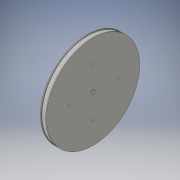
# Autodesk Inventor part: Wheel
Saved by Autodesk Inventor 2016 (Build 200138000, 138)
## iProperties
Created: 2016-10-07
Part Number: Wheel
Material: Generic
Document SubType Name: Modeling
Designer: sheehm
Density: 1 g/cm^3
Appearance: Default
Author: sheehm
Autodesk Inventor part; units mm, degrees
ref_plane "YZ Plane" through (0, 0, 0) normal (1, 0, 0) x (0, 1, 0)
ref_plane "XZ Plane" through (0, 0, 0) normal (0, 1, 0) x (-1, 0, 0)
ref_plane "XY Plane" through (0, 0, 0) normal (0, 0, 1) x (1, 0, 0)
sketch "Sketch1" plane through (0, 0, 0) normal (1, 0, 0) x (0, 1, 0)
  circle A0 centre (0, 0) radius 30.48
  dimension "d0" = 60.96
  constraints: 1 centre point, 1 coincident
  measures "d0" diameter of A0
extrude "Extrusion1" add sketch "Sketch1" along normal blind 3.048
sketch "Sketch2" plane through (3.048, 0, 0) normal (1, 0, 0) x (0, 0, -1)
  circle A0 centre (0, 0) radius 30.9541
  constraints: 1 centre point, 1 coincident
extrude "Extrusion2" add sketch "Sketch2" along normal blind 0.508
sketch "Sketch3" plane through (0, 0, 0) normal (-1, 0, 0) x (0, 0, 1)
  circle A0 centre (0, 0) radius 30.9541
  constraints: 1 centre point, 1 coincident
extrude "Extrusion3" add sketch "Sketch3" along normal blind 0.508
sketch "Sketch4" plane through (3.556, 0, 0) normal (1, 0, 0) x (0, 0, -1)
  circle A0 centre (0, 0) radius 1.3
  dimension "d7" = 2.6
  constraints: 1 centre point, 1 coincident
  measures "d7" diameter of A0
hole "Hole1" at (3.556, 0, 0) direction (-1, 0, 0) diameter 2.6 end through all
sketch "Sketch5" plane through (3.556, 0, 0) normal (1, 0, 0) x (0, 0, -1)
  circle A0 centre (0, 0) radius 1.3 projected
  circle A1 centre (-16.2, 0) radius 0.5
  circle A2 centre (0, 16.2) radius 0.5
  circle A3 centre (16.2, 0) radius 0.5
  circle A4 centre (0, -16.2) radius 0.5
  dimension "d19" = 1
  dimension "d20" = 1
  dimension "d21" = 1
  dimension "d22" = 1
  constraints: 4 centre point
  measures "d19" diameter of A1
  measures "d20" diameter of A2
  measures "d21" diameter of A3
  measures "d22" diameter of A4
hole "Hole2" at (3.556, 16.2, 0) at (3.556, -16.2, 0) at (3.556, 0, -16.2) at (3.556, 0, 16.2) direction (-1, 0, 0) diameter 1 end through all
sketch "Sketch6" plane through (-0.508, 0, 0) normal (-1, 0, 0) x (0, 0, 1)
  arc A0 (1.5256, -7.6067) -> (-1.5256, -7.6067) centre (0, -8.5367) ccw
  line L0 (1.5256, -7.6067) -> (10.0877, -14.0155)
  arc A1 (10.0877, -14.0155) -> (14.0155, -10.0877) centre (11.7691, -11.7691) ccw
  line L1 (14.0155, -10.0877) -> (7.6067, -1.5256)
  arc A2 (7.6067, 1.5256) -> (7.6067, -1.5256) centre (8.5367, 0) ccw
  line L2 (7.6067, 1.5256) -> (14.0155, 10.0877)
  arc A3 (14.0155, 10.0877) -> (10.0877, 14.0155) centre (11.7691, 11.7691) ccw
  line L3 (10.0877, 14.0155) -> (1.5256, 7.6067)
  arc A4 (-1.5256, 7.6067) -> (1.5256, 7.6067) centre (0, 8.5367) ccw
  line L4 (-1.5256, 7.6067) -> (-10.0877, 14.0155)
  arc A5 (-10.0877, 14.0155) -> (-14.0155, 10.0877) centre (-11.7691, 11.7691) ccw
  line L5 (-14.0155, 10.0877) -> (-7.6067, 1.5256)
  arc A6 (-7.6067, -1.5256) -> (-7.6067, 1.5256) centre (-8.5367, 0) ccw
  line L6 (-7.6067, -1.5256) -> (-14.0155, -10.0877)
  arc A7 (-14.0155, -10.0877) -> (-10.0877, -14.0155) centre (-11.7691, -11.7691) ccw
  line L7 (-10.0877, -14.0155) -> (-1.5256, -7.6067)
  circle A8 centre (12.339, -12.339) radius 0.75
  circle A9 centre (9.8641, -9.8641) radius 0.75
  circle A10 centre (7.3893, -7.3893) radius 0.75
  circle A11 centre (4.9144, -4.9144) radius 0.75
  circle A12 centre (12.339, 12.339) radius 0.75
  circle A13 centre (9.8641, 9.8641) radius 0.75
  circle A14 centre (7.3893, 7.3893) radius 0.75
  circle A15 centre (4.9144, 4.9144) radius 0.75
  circle A16 centre (-12.339, 12.339) radius 0.75
  circle A17 centre (-9.8641, 9.8641) radius 0.75
  circle A18 centre (-7.3893, 7.3893) radius 0.75
  circle A19 centre (-4.9144, 4.9144) radius 0.75
  circle A20 centre (-12.339, -12.339) radius 0.75
  circle A21 centre (-9.8641, -9.8641) radius 0.75
  circle A22 centre (-7.3893, -7.3893) radius 0.75
  circle A23 centre (-4.9144, -4.9144) radius 0.75
  circle A24 centre (0, 0) radius 3.6
  point P0 (0, 0)
  constraints: 25 centre point, 16 end point, 16 point on circle
extrude "Extrusion4" cut sketch "Sketch6" against normal blind 2.1844 contours A0 L7 A7 L6 A6 L5 A5 L4 A4 L3 A3 L2 A2 L1 A1 L0 | A8 | A9 | A10 | A11 | A12 | A13 | A14 | A15 | A16 | A17 | A18 | A19 | A20 | A21 | A22 | A23 | A24
body "Solid1"
